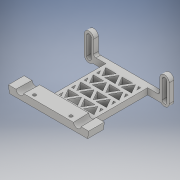
# Autodesk Inventor part: Bar_Mount_Bottom
Saved by Autodesk Inventor 2019 (Build 230136000, 136)
## iProperties
Created: 2019-08-14
Part Number: Bar_Mount_Bottom
Material: Generic
Document SubType Name: Modeling
Designer: steve
Density: 1 g/cm^3
Appearance: Default
Author: steve
Autodesk Inventor part; units mm, degrees
ref_plane "YZ Plane" through (0, 0, 0) normal (1, 0, 0) x (0, 1, 0)
ref_plane "XZ Plane" through (0, 0, 0) normal (0, 1, 0) x (-1, 0, 0)
sketch "Sketch1" plane through (0, 0, 0) normal (0, 0, 1) x (1, 0, 0)
  line L0 (75, -6.6976) -> (-75, -6.6976)
  line L1 (-75, -6.6976) -> (-77.0141, 6.8774)
  line L2 (-77.0141, 6.8774) -> (-61.6574, 6.8774)
  line L3 (77.0141, 6.8774) -> (75, -6.6976)
  line L4 (75, -6.6976) -> (-77.0141, 6.8774) construction
  line L5 (-75, -6.6976) -> (77.0141, 6.8774) construction
  line L6 (-77.1625, 7.8774) -> (77.8086, 7.8774) construction
  arc A0 (-46.9426, 6.8774) -> (-61.6574, 6.8774) centre (-54.3, 7.8774) ccw construction
  arc A1 (47.8105, 4.2695) -> (61.6574, 6.8774) centre (54.3, 7.8774) ccw
  line L7 (46.9426, 6.8774) -> (61.6574, 6.8774) construction
  line L8 (61.6574, 6.8774) -> (77.0141, 6.8774)
  arc A2 (46.9426, 6.8774) -> (47.8105, 4.2695) centre (54.3, 7.8774) ccw
  arc A3 (61.6574, 6.8774) -> (46.9426, 6.8774) centre (54.3, 7.8774) ccw construction
  line L9 (-61.6574, 6.8774) -> (-46.9426, 6.8774) construction
  line L10 (-46.9426, 6.8774) -> (46.9426, 6.8774)
  arc A4 (-47.8105, 4.2695) -> (-46.9426, 6.8774) centre (-54.3, 7.8774) ccw
  arc A5 (-61.3261, 5.4765) -> (-47.8105, 4.2695) centre (-54.3, 7.8774) ccw
  arc A6 (-61.6574, 6.8774) -> (-61.3261, 5.4765) centre (-54.3, 7.8774) ccw
  point P0 (0, 0)
  dimension "d0" = 1
  dimension "d1" = 14.85
  dimension "d2" = 54.3
  dimension "d3" = 108.6
  dimension "d5" = 150
  dimension "d6" = 22.7141
  dimension "d7" = 22.7141
  dimension "d8" = 14.575
  constraints: 22 end point, 15 point on circle, 8 point on line, 7 centre point, 6 horizontal, 5 parallel, 1 equal radius
  measures "d0" distance between parallel lines of L6 L2
  measures "d1" diameter of A0
  measures "d2" horizontal distance of point (0, 0) A0.centre
  measures "d3" distance of A1.centre A0.centre
  measures "d5" distance of L0.start L0.end
  measures "d6" horizontal distance of L1.end A0.centre
  measures "d7" horizontal distance of L3.start A1.centre
  measures "d8" distance from line of A0.centre L0
ref_plane "Work Plane1" through (0, 0, 30) normal (0, 0, 1) x (1, 0, 0)
sketch "Sketch2" plane through (0, 0, 30) normal (0, 0, 1) x (1, 0, 0)
  line L0 (75, -6.6976) -> (-75, -6.6976) projected
  line L1 (-75, -6.6976) -> (-77.0141, 6.8774) projected
  line L2 (77.0141, 6.8774) -> (75, -6.6976) projected
  line L3 (62.5574, 6.8774) -> (77.0141, 6.8774)
  line L4 (-47.8426, 6.8774) -> (47.8426, 6.8774)
  line L5 (-77.0141, 6.8774) -> (-62.5574, 6.8774)
  line L6 (-77.1625, 7.8774) -> (77.8086, 7.8774) construction
  arc A0 (-62.5574, 6.8774) -> (-47.8426, 6.8774) centre (-55.2, 7.8774) ccw
  arc A1 (47.8426, 6.8774) -> (62.5574, 6.8774) centre (55.2, 7.8774) ccw
  point P0 (0, 0)
  dimension "d10" = 7.425
  dimension "d11" = 110.4
  dimension "d12" = 55.2
  constraints: 6 end point, 4 point on circle, 2 centre point, 2 collinear, 2 point on line, 1 equal radius
  measures "d10" radius of A0
  measures "d11" distance of A1.centre A0.centre
  measures "d12" horizontal distance of A0.centre point (0, 0)
loft "Loft1" add profiles "Sketch1", "Sketch2"
sketch "Sketch8" plane through (-75, -6.6976, 0) normal (0, -1, 0) x (1, 0, 0)
  circle A0 centre (110, 22) radius 3
  circle A1 centre (40, 22) radius 3
  point P0 (75, 0)
  dimension "d31" = 35
  dimension "d32" = 35
  dimension "d33" = 22
  dimension "d34" = 22
  dimension "d35" = 6
  constraints: 2 centre point, 1 equal radius
  measures "d31" horizontal distance of point (75, 0) A0.centre
  measures "d32" horizontal distance of point (75, 0) A1.centre
  measures "d33" vertical distance of point (75, 0) A0.centre
  measures "d34" vertical distance of point (75, 0) A1.centre
  measures "d35" diameter of A0
extrude "Extrusion3" cut sketch "Sketch8" against normal through all
sketch "Sketch9" plane through (-75, -6.6976, 0) normal (0, -1, 0) x (1, 0, 0)
  circle A0 centre (110, 22) radius 3 projected
  circle A1 centre (40, 22) radius 3 projected
  line L0 (107.1132, 27) -> (112.8868, 27)
  line L1 (112.8868, 27) -> (115.7735, 22)
  line L2 (115.7735, 22) -> (112.8868, 17)
  line L3 (112.8868, 17) -> (107.1132, 17)
  line L4 (107.1132, 17) -> (104.2265, 22)
  line L5 (104.2265, 22) -> (107.1132, 27)
  line L6 (37.1132, 27) -> (42.8868, 27)
  line L7 (42.8868, 27) -> (45.7735, 22)
  line L8 (45.7735, 22) -> (42.8868, 17)
  line L9 (42.8868, 17) -> (37.1132, 17)
  line L10 (37.1132, 17) -> (34.2265, 22)
  line L11 (34.2265, 22) -> (37.1132, 27)
  point P0 (75, 0)
  dimension "d38" = 10
  constraints: 24 end point, 2 coincident, 2 horizontal, 1 collinear, 26 other
  measures "d38" distance between parallel lines of L0 L3
extrude "Extrusion4" cut sketch "Sketch9" against normal blind 5 and the other way blind 100
sketch "Sketch10" plane through (75, -6.6976, 0) normal (0, 0, -1) x (-1, 0, 0)
  line L0 (115, -7.85) -> (35, -7.85)
  line L1 (35, -7.85) -> (35, -19.85)
  line L2 (35, -19.85) -> (115, -19.85)
  line L3 (115, -19.85) -> (115, -7.85)
  arc A0 (12.4426, 13.575) -> (27.1574, 13.575) centre (19.8, 14.575) ccw projected
  point P0 (75, -7.85)
  dimension "d43" = 40
  dimension "d44" = 40
  dimension "d45" = 12
  dimension "d104" = 7.425
  dimension "d105" = 15
  constraints: 8 end point, 2 parallel, 1 horizontal, 1 midpoint, 1 perpendicular
  measures "d43" distance from line of point (75, -7.85) L1
  measures "d44" distance from line of point (75, -7.85) L3
  measures "d45" distance between parallel lines of L0 L2
  measures "d104" radius of A0
  measures "d105" distance edge to line of A0 L0
extrude "Extrusion5" add sketch "Sketch10" along normal blind 120
sketch "Sketch11" plane through (75, -6.6976, -120) normal (0, 0, -1) x (-1, 0, 0)
  arc A0 (7, -13.85) -> (-2, -13.85) centre (2.5, -13.85) ccw
  arc A1 (152, -13.85) -> (143, -13.85) centre (147.5, -13.85) ccw
  arc A2 (9.2082, -7.85) -> (-6.5, -13.85) centre (2.5, -13.85) ccw
  line L0 (6.0389, -13.85) -> (-6.5, -13.85) construction
  line L1 (4.1756, -13.85) -> (171.8785, -13.85) construction
  line L2 (9.2082, -7.85) -> (140.7918, -7.85)
  line L3 (115, -7.85) -> (35, -7.85) projected
  line L4 (156.5, -33.85) -> (156.5, -13.85)
  line L5 (152, -33.85) -> (152, -13.85)
  line L6 (143, -33.85) -> (143, -13.85)
  line L7 (138.5, -33.85) -> (138.5, -5.3)
  arc A3 (156.5, -13.85) -> (140.7918, -7.85) centre (147.5, -13.85) ccw
  line L8 (138.5, -5.3) -> (11.5, -5.3)
  arc A4 (138.5, -33.85) -> (156.5, -33.85) centre (147.5, -33.85) ccw
  arc A5 (143, -33.85) -> (152, -33.85) centre (147.5, -33.85) ccw
  line L9 (-6.5, -33.85) -> (-6.5, -13.85)
  line L10 (0, 0) -> (150, 0) projected
  line L11 (7, -33.85) -> (7, -13.85)
  line L12 (11.5, -33.85) -> (11.5, -5.3)
  arc A6 (-2, -33.85) -> (7, -33.85) centre (2.5, -33.85) ccw
  arc A7 (-6.5, -33.85) -> (11.5, -33.85) centre (2.5, -33.85) ccw
  line L13 (-2, -33.85) -> (-2, -13.85)
  point P0 (75, 6.6976)
  point P1 (75, -7.85)
  point P2 (35, -7.85)
  point P3 (35, 0)
  dimension "d48" = 145
  dimension "d49" = 9
  dimension "d60" = 6
  dimension "d61" = 5.3
  dimension "d62" = 4.5
  dimension "d63" = 4.5
  dimension "d64" = 0
  dimension "d66" = 4.5
  dimension "d67" = 20
  dimension "d70" = 72.5
  constraints: 24 end point, 16 point on circle, 8 centre point, 8 tangent, 7 point on line, 6 vertical, 3 coincident, 3 equal radius, 3 parallel, 2 horizontal, 2 perpendicular, 1 midpoint, 2 other
  measures "d48" distance of A0.centre A1.centre
  measures "d49" diameter of A0
  measures "d61" distance between parallel lines of L10 L8
  measures "d62" distance between parallel lines of L6 L7
  measures "d63" distance between parallel lines of L4 L5
  measures "d64" distance of A5.centre A4.centre
  measures "d66" distance between parallel lines of L11 L12
  measures "d67" distance of A4.centre A3.centre
  measures "d70" horizontal distance of A1.centre point (75, -7.85)
extrude "Extrusion6" [suppressed]
sketch "Sketch12" plane through (75, -6.6976, -120) normal (0, 0, -1) x (-1, 0, 0)
  arc A0 (-2, -13.85) -> (7, -13.85) centre (2.5, -13.85) ccw
  arc A1 (143, -13.85) -> (152, -13.85) centre (147.5, -13.85) ccw
  arc A2 (-6.4996, -13.85) -> (9.2077, -19.85) centre (2.5, -13.85) ccw
  line L0 (9.2077, -19.85) -> (140.7923, -19.85)
  line L1 (156.4996, 21.15) -> (156.4996, -13.85)
  line L2 (138.5004, 21.15) -> (138.5004, -7.85)
  arc A3 (140.7923, -19.85) -> (156.4996, -13.85) centre (147.5, -13.85) ccw
  line L3 (138.5004, -7.85) -> (11.4996, -7.85)
  arc A4 (156.4996, 21.15) -> (138.5004, 21.15) centre (147.5, 21.15) ccw
  arc A5 (152, 21.15) -> (143, 21.15) centre (147.5, 21.15) ccw
  line L4 (-6.4996, 21.15) -> (-6.4996, -13.85)
  line L5 (11.4996, 21.15) -> (11.4996, -7.85)
  arc A6 (7, 21.15) -> (-2, 21.15) centre (2.5, 21.15) ccw
  arc A7 (11.4996, 21.15) -> (-6.4996, 21.15) centre (2.5, 21.15) ccw
  line L6 (7, 21.15) -> (7, -13.85)
  line L7 (-2, 21.15) -> (-2, -13.85)
  line L8 (143, 21.15) -> (143, -13.85)
  line L9 (152, 21.15) -> (152, -13.85)
  line L10 (115, -7.85) -> (35, -7.85) projected
  point P0 (75, 6.6976)
  point P1 (75, -7.85)
  point P2 (35, -7.85)
  dimension "d90" = 12
  dimension "d91" = 4.5
  dimension "d92" = 6
  dimension "d93" = 35
  dimension "d94" = 4.4996
  dimension "d95" = 145
  constraints: 20 end point, 16 point on circle, 14 tangent, 8 centre point, 7 vertical, 4 parallel, 3 coincident, 3 equal radius, 2 perpendicular, 1 midpoint, 2 other
  measures "d90" distance between parallel lines of L0 L3
  measures "d91" radius of A0
  measures "d92" distance from line of A0.centre L3
  measures "d93" distance of A0.centre A6.centre
  measures "d94" distance between parallel lines of L6 L5
  measures "d95" distance of A1.centre A0.centre
extrude "Extrusion7" add sketch "Sketch12" along normal blind 9
sketch "Sketch13" plane through (-75, -6.6976, 30) normal (0, -1, 0) x (1, 0, 0)
  line L0 (150, -30) -> (0, -30) projected
  line L1 (35, -30) -> (115, -30)
  line L2 (115, -30) -> (115, -20)
  line L3 (115, -20) -> (35, -20)
  line L4 (35, -20) -> (35, -30)
  point P0 (75, -30)
  dimension "d100" = 10
  constraints: 8 end point, 2 parallel, 1 horizontal, 1 perpendicular
  measures "d100" distance of L1.end L2.end
extrude "Extrusion8" add sketch "Sketch13" along normal blind 20
fillet "Fillet1" radius 8.25 1 edges at (0, -14.5476, 0)
fillet "Fillet2" radius 4.25 2 edges at (-63.5004, -14.5476, -124.5) (63.5004, -14.5476, -124.5)
sketch "Sketch14" plane through (-40, -14.5476, -8.25) normal (0, 1, 0) x (1, 0, 0)
  line L0 (47.8426, 15.6529) -> (37.8426, 32.9734)
  line L1 (37.8426, 32.9734) -> (57.8426, 32.9734)
  line L2 (57.8426, 32.9734) -> (47.8426, 15.6529)
  line L3 (73.5278, 15.5) -> (53.5278, 15.5)
  line L4 (53.5278, 15.5) -> (63.5278, 32.8205)
  line L5 (63.5278, 32.8205) -> (73.5278, 15.5)
  line L6 (80, 0) -> (0, 0) projected
  line L7 (80, 0) -> (80, 111.75) projected
  line L8 (16.4722, 15.6529) -> (6.4722, 32.9734)
  line L9 (6.4722, 32.9734) -> (26.4722, 32.9734)
  line L10 (26.4722, 32.9734) -> (16.4722, 15.6529)
  line L11 (42.1574, 15.5) -> (22.1574, 15.5)
  line L12 (22.1574, 15.5) -> (32.1574, 32.8205)
  line L13 (32.1574, 32.8205) -> (42.1574, 15.5)
  line L14 (47.8426, 39.6529) -> (37.8426, 56.9734)
  line L15 (37.8426, 56.9734) -> (57.8426, 56.9734)
  line L16 (57.8426, 56.9734) -> (47.8426, 39.6529)
  line L17 (73.5278, 39.5) -> (53.5278, 39.5)
  line L18 (53.5278, 39.5) -> (63.5278, 56.8205)
  line L19 (63.5278, 56.8205) -> (73.5278, 39.5)
  line L20 (16.4722, 39.6529) -> (6.4722, 56.9734)
  line L21 (6.4722, 56.9734) -> (26.4722, 56.9734)
  line L22 (26.4722, 56.9734) -> (16.4722, 39.6529)
  line L23 (42.1574, 39.5) -> (22.1574, 39.5)
  line L24 (22.1574, 39.5) -> (32.1574, 56.8205)
  line L25 (32.1574, 56.8205) -> (42.1574, 39.5)
  line L26 (47.8426, 63.6529) -> (37.8426, 80.9734)
  line L27 (37.8426, 80.9734) -> (57.8426, 80.9734)
  line L28 (57.8426, 80.9734) -> (47.8426, 63.6529)
  line L29 (73.5278, 63.5) -> (53.5278, 63.5)
  line L30 (53.5278, 63.5) -> (63.5278, 80.8205)
  line L31 (63.5278, 80.8205) -> (73.5278, 63.5)
  line L32 (16.4722, 63.6529) -> (6.4722, 80.9734)
  line L33 (6.4722, 80.9734) -> (26.4722, 80.9734)
  line L34 (26.4722, 80.9734) -> (16.4722, 63.6529)
  line L35 (42.1574, 63.5) -> (22.1574, 63.5)
  line L36 (22.1574, 63.5) -> (32.1574, 80.8205)
  line L37 (32.1574, 80.8205) -> (42.1574, 63.5)
  line L38 (47.8426, 87.6529) -> (37.8426, 104.9734)
  line L39 (37.8426, 104.9734) -> (57.8426, 104.9734)
  line L40 (57.8426, 104.9734) -> (47.8426, 87.6529)
  line L41 (73.5278, 87.5) -> (53.5278, 87.5)
  line L42 (53.5278, 87.5) -> (63.5278, 104.8205)
  line L43 (63.5278, 104.8205) -> (73.5278, 87.5)
  line L44 (16.4722, 87.6529) -> (6.4722, 104.9734)
  line L45 (6.4722, 104.9734) -> (26.4722, 104.9734)
  line L46 (26.4722, 104.9734) -> (16.4722, 87.6529)
  line L47 (42.1574, 87.5) -> (22.1574, 87.5)
  line L48 (22.1574, 87.5) -> (32.1574, 104.8205)
  line L49 (32.1574, 104.8205) -> (42.1574, 87.5)
  line L50 (73.5278, 32.9734) -> (73.5278, 25.5)
  line L51 (73.5278, 32.9734) -> (69.2131, 32.9734)
  line L52 (69.2131, 32.9734) -> (73.5278, 25.5)
  line L53 (73.5278, 56.9734) -> (69.2131, 56.9734)
  line L54 (73.5278, 56.9734) -> (73.5278, 49.5)
  line L55 (69.2131, 56.9734) -> (73.5278, 49.5)
  line L56 (73.5278, 80.9734) -> (69.2131, 80.9734)
  line L57 (73.5278, 80.9734) -> (73.5278, 73.5)
  line L58 (69.2131, 80.9734) -> (73.5278, 73.5)
  line L59 (73.5278, 104.9734) -> (69.2131, 104.9734)
  line L60 (73.5278, 104.9734) -> (73.5278, 97.5)
  line L61 (69.2131, 104.9734) -> (73.5278, 97.5)
  line L62 (6.4722, 15.5) -> (6.4722, 22.9734)
  line L63 (6.4722, 22.9734) -> (10.7869, 15.5)
  line L64 (10.7869, 15.5) -> (6.4722, 15.5)
  line L65 (6.4722, 39.5) -> (6.4722, 46.9734)
  line L66 (6.4722, 46.9734) -> (10.7869, 39.5)
  line L67 (10.7869, 39.5) -> (6.4722, 39.5)
  line L68 (6.4722, 63.5) -> (6.4722, 70.9734)
  line L69 (6.4722, 70.9734) -> (10.7869, 63.5)
  line L70 (10.7869, 63.5) -> (6.4722, 63.5)
  line L71 (6.4722, 87.5) -> (6.4722, 94.9734)
  line L72 (6.4722, 94.9734) -> (10.7869, 87.5)
  line L73 (10.7869, 87.5) -> (6.4722, 87.5)
  point P0 (40, -8.25)
  point P1 (73.5278, 87.5)
  dimension "d109" = 20
  dimension "d110" = 5
  dimension "d111" = 25.6852
  dimension "d112" = 5.6852
  dimension "d115" = 31.3704
  dimension "d118" = 24
  dimension "d121" = 67.0557
  dimension "d122" = 80
  dimension "d123" = 6.4722
  dimension "d124" = 5
  dimension "d125" = 15.5
  dimension "d128" = 24
  dimension "d133" = 5
  dimension "d136" = 24
  constraints: 144 end point, 8 point on line, 5 equal length, 5 vertical, 4 horizontal, 2 collinear, 2 parallel, 1 perpendicular, 126 other
  measures "d109" distance of L3.start L3.end
  measures "d110" distance between parallel lines of L2 L4
  measures "d111" horizontal distance of L0.start L3.start
  measures "d112" horizontal distance of L3.end L0.start
  measures "d115" distance of L0.start L8.start
  measures "d118" distance of L0.start L14.start
  measures "d121" horizontal distance of L8.end L3.start
  measures "d122" distance of L6.start L6.end
  measures "d123" distance from line of L7 L3.start
  measures "d124" distance between parallel lines of L5 L52
  measures "d125" distance between parallel lines of L6 L11
  measures "d128" distance of L50.end L54.end
  measures "d133" distance between parallel lines of L8 L63
  measures "d136" distance of L62.start L65.start
extrude "Extrusion9" cut sketch "Sketch14" against normal up to next
equation "\"d2\" = 0.5 * d3"
equation "\"d7\" = d6"
equation "\"d10\" = 0.5 * d1"
equation "\"d12\" = 0.5 * d11"
equation "\"d32\" = d31"
equation "\"d34\" = d33"
equation "\"d44\" = d43"
equation "\"d63\" = d62"
equation "\"d66\" = d62"
body "Solid1"
